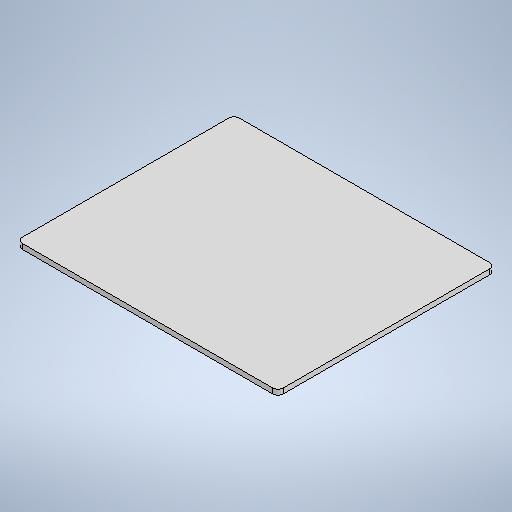
# Autodesk Inventor part: ANP 1424 FDS diam way cup
Saved by Autodesk Inventor 2025 (Build 290162010, 162A)
## iProperties
Created: 2025-06-24
Part Number: ANP 1424 FDS diam way cup
Material: Stainless Steel
Document SubType Name: Sheet Metal
Designer: admin
Mass: 14.3451 g
Surface Area: 20.2627 cm^2
Volume: 1.79313 cm^3
Density: 8 g/cm^3
Flat Pattern Width: 10.1 cm
Flat Pattern Length: 8.4 cm
Flat Pattern Area: 84.84 cm^2
Sheet Metal Rule: AISI304 2mm Die16
Sheet Metal Width: 101,000 mm
Sheet Metal Length: 84,000 mm
Sheet Metal Area: 8484,000 mm^2
Appearance: Default
Author: user
Autodesk Inventor part; units mm, degrees
ref_plane "YZ Plane" through (0, 0, 0) normal (1, 0, 0) x (0, 1, 0)
ref_plane "XZ Plane" through (0, 0, 0) normal (0, 1, 0) x (-1, 0, 0)
ref_plane "XY Plane" through (0, 0, 0) normal (0, 0, 1) x (1, 0, 0)
sketch "Sketch1" plane through (0, 0, 0) normal (0, 0, 1) x (1, 0, 0)
  line L0 (-50.5, -42) -> (50.5, -42)
  line L1 (50.5, -42) -> (50.5, 42)
  line L2 (50.5, 42) -> (-50.5, 42)
  line L3 (-50.5, 42) -> (-50.5, -42)
  line L4 (-50.5, -42) -> (50.5, 42) construction
  line L5 (50.5, -42) -> (-50.5, 42) construction
  point P0 (0, 0)
  dimension "d154" = 101
  dimension "d155" = 84
  measures "d154" distance of L1.end L2.end
  measures "d155" distance of L0.end L1.end
extrude "Plate5" add sketch "Sketch1" along normal blind 2
fillet "Corner Round1" radius 2 4 edges at (50.5, 42, 1) (50.5, -42, 1) (-50.5, -42, 1) (-50.5, 42, 1)
sketch "Sketch11" plane through (-50.5, -22, -28) normal (1, 0, 0) x (0, 0, -1)
  line L0 (-25.25, 44) -> (-25.25, 0) construction
  line L1 (0, 0) -> (-25.25, 0) construction
  line L2 (0, 0) -> (0, 44) construction
  line L3 (0, 44) -> (-25.25, 44) construction
  circle A0 centre (-10, 22) radius 5.5
  point P0 (-28, 22)
  point P1 (0, 22)
  dimension "d192" = 11
  dimension "d193" = 10
  constraints: 1 centre point, 1 horizontal alignment, 1 midpoint
  measures "d192" diameter of A0
  measures "d193" distance from line of A0.centre L2
cut "Cut3" [suppressed]
feature "Corner Round3" [suppressed]
sketch "Sketch10" plane through (-52.5, 40, 2) normal (1, 0, 0) x (0, 1, 0)
  line L0 (-80, 0) -> (0, 0)
  line L1 (0, 0) -> (0, -30)
  line L2 (0, -30) -> (-80, -30)
  line L3 (-80, -30) -> (-80, 0)
  constraints: 8 end point
body "Solid3"
